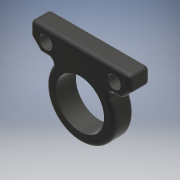
# Autodesk Inventor part: proxymity_holder_v2
Saved by Autodesk Inventor 2018 (Build 220112000, 112)
## iProperties
Created: 2018-07-23
Part Number: proxymity_holder_v2
Material: ABS Plastic
Document SubType Name: Modeling
Designer: Z. Deniz
Density: 1.06 g/cm^3
Appearance: Smooth - White
Author: Z. Deniz
Autodesk Inventor part; units mm, degrees
ref_plane "YZ Plane" through (0, 0, 0) normal (1, 0, 0) x (0, 1, 0)
ref_plane "XZ Plane" through (0, 0, 0) normal (0, 1, 0) x (-1, 0, 0)
ref_plane "XY Plane" through (0, 0, 0) normal (0, 0, 1) x (1, 0, 0)
sketch "Sketch1" plane through (0, 0, 0) normal (0, 1, 0) x (-1, 0, 0)
  circle A0 centre (0, 0) radius 6
  circle A1 centre (0, 0) radius 8.5
  line L0 (12.5, 12) -> (-12.5, 12)
  line L1 (-12.5, 12) -> (-12.5, 6)
  line L2 (-12.5, 6) -> (12.5, 6)
  line L3 (12.5, 6) -> (12.5, 12)
  line L4 (12.5, 9) -> (-12.5, 9) construction
  circle A2 centre (8.5, 9) radius 1.625
  circle A3 centre (-8.5, 9) radius 1.625
  dimension "d0" = 12
  dimension "d1" = 17
  dimension "d2" = 25
  dimension "d3" = 6
  dimension "d4" = 12.5
  dimension "d5" = 3.25
  dimension "d6" = 3.25
  dimension "d7" = 17
  dimension "d8" = 4
  constraints: 10 end point, 4 centre point, 2 coincident, 2 midpoint, 2 parallel, 2 point on line, 1 horizontal, 1 perpendicular, 1 tangent
  measures "d0" diameter of A0
  measures "d1" diameter of A1
  measures "d2" distance of L0.start L0.end
  measures "d3" distance of L0.end L1.end
  measures "d4" distance from line of L3 point (0, 0)
  measures "d5" diameter of A2
  measures "d6" diameter of A3
  measures "d7" distance of A3.centre A2.centre
  measures "d8" distance from line of L3 A2.centre
extrude "Extrusion1" add sketch "Sketch1" along normal blind 5
chamfer "Chamfer2" distance 2.5 angle 45 2 edges at (-12.5, 2.5, 6) (12.5, 2.5, 6)
fillet "Fillet3" radius 1 24 edges at (8.0104, 0, 6) (11.25, 0, 7.25) (12.5, 0, 10.25) (0, 0, 12) (-12.5, 0, 10.25) (-8.0104, 0, 6) (-10, 2.5, 6) (-12.5, 5, 10.25) (-12.5, 2.5, 8.5) (-11.25, 5, 7.25) (-8.0104, 5, 6) (-11.25, 0, 7.25) (-6.0208, 2.5, 6) (6.0208, 2.5, 6) (0, 0, -8.5) (0, 5, -8.5) (8.0104, 5, 6) (10, 2.5, 6) (11.25, 5, 7.25) (12.5, 5, 10.25) (0, 5, 12) (-12.5, 2.5, 12) (12.5, 2.5, 8.5) (12.5, 2.5, 12)
equation "\"d4\" = 0.5 * d2"
equation "\"d8\" = -0.5 * d7 + 0.5 * d2"
body "Solid1"
